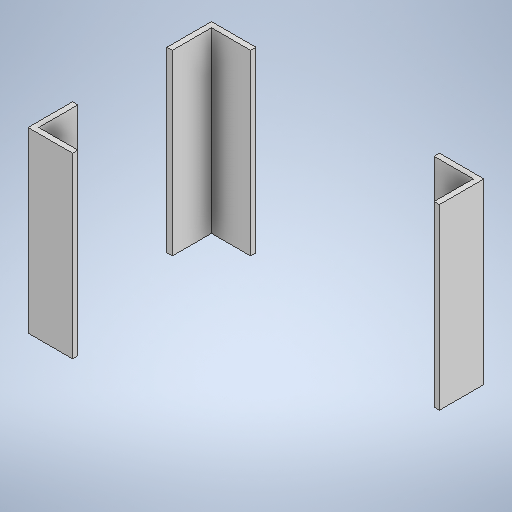
# Autodesk Inventor part: slot pillars
Saved by Autodesk Inventor 2025.2 (Build 292293000, 293)
## iProperties
Created: 2025-02-04
Part Number: slot pillars
Material: Generic
Document SubType Name: Modeling
Designer: nandu
Density: 1 g/cm^3
Appearance: Default
Author: nandu
Autodesk Inventor part; units mm, degrees
ref_plane "YZ Plane" through (0, 0, 0) normal (1, 0, 0) x (0, 1, 0)
ref_plane "XZ Plane" through (0, 0, 0) normal (0, 1, 0) x (-1, 0, 0)
ref_plane "XY Plane" through (0, 0, 0) normal (0, 0, 1) x (1, 0, 0)
sketch "Sketch1" plane through (0, 0, 0) normal (0, 1, 0) x (-1, 0, 0)
  line L0 (0, -100) -> (0, -103)
  line L1 (0, -103) -> (25, -103)
  line L2 (25, -103) -> (25, -100)
  line L3 (25, -100) -> (3, -100)
  line L4 (3, -100) -> (3, -78)
  line L5 (3, -78) -> (0, -78)
  line L6 (0, -78) -> (0, -100)
  line L7 (150, -100) -> (128, -100)
  line L8 (128, -100) -> (128, -103)
  line L9 (128, -103) -> (153, -103)
  line L10 (153, -103) -> (153, -78)
  line L11 (153, -78) -> (150, -78)
  line L12 (150, -78) -> (150, -100)
  line L13 (150, -3) -> (150, -25)
  line L14 (150, -25) -> (153, -25)
  line L15 (153, -25) -> (153, 0)
  line L16 (153, 0) -> (128, 0)
  line L17 (128, 0) -> (128, -3)
  line L18 (128, -3) -> (150, -3)
  line L19 (25, -103) -> (25, -100)
  line L20 (128, -100) -> (128, -103)
  line L21 (153, -78) -> (150, -78)
  line L22 (150, -25) -> (153, -25)
  line L23 (150, -3) -> (147, -3)
  line L24 (147, -100) -> (150, -100)
  line L25 (147, -100) -> (147, -97)
  line L26 (3, -97) -> (3, -100)
  point P0 (0, 0)
  dimension "d0" = 3
  dimension "d1" = 25
  dimension "d2" = 3
  dimension "d3" = 22
  dimension "d4" = 22
  dimension "d5" = 3
  dimension "d6" = 22
  dimension "d7" = 3
  dimension "d8" = 25
  dimension "d9" = 25
  dimension "d10" = 3
  dimension "d11" = 22
  dimension "d12" = 3
  dimension "d13" = 25
  dimension "d14" = 25
  dimension "d15" = 3
  dimension "d18" = 3
  dimension "d19" = 3
  constraints: 54 end point, 10 perpendicular, 5 parallel, 4 horizontal, 2 point on line, 2 vertical
  measures "d0" distance of L0.start L0.end
  measures "d1" distance of L0.end L1.end
  measures "d2" distance of L1.end L2.end
  measures "d3" distance of L2.end L3.end
  measures "d4" distance of L3.end L4.end
  measures "d5" distance of L4.end L5.end
  measures "d6" distance of L7.start L7.end
  measures "d7" distance of L7.end L8.end
  measures "d8" distance of L8.end L9.end
  measures "d9" distance of L9.end L10.end
  measures "d10" distance of L10.end L11.end
  measures "d11" distance of L13.start L13.end
  measures "d12" distance of L13.end L14.end
  measures "d13" distance of L14.end L15.end
  measures "d14" distance of L15.end L16.end
  measures "d15" distance of L16.end L17.end
  measures "d18" distance of L24.end L24.start
  measures "d19" distance of L25.end L25.start
extrude "Extrusion1" add sketch "Sketch1" along normal blind 100
body "Solid1"
